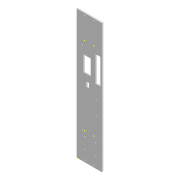
# Autodesk Inventor part: top of drivetrain 2
Saved by Autodesk Inventor 2020 (Build 240168000, 168)
## iProperties
Created: 2020-03-07
Part Number: top of drivetrain 2
Material: Generic
Document SubType Name: Modeling
Designer: jackm
Density: 1 g/cm^3
Appearance: Default
Author: jackm
Autodesk Inventor part; units mm, degrees
ref_plane "YZ Plane" through (0, 0, 0) normal (1, 0, 0) x (0, 1, 0)
ref_plane "XZ Plane" through (0, 0, 0) normal (0, 1, 0) x (-1, 0, 0)
ref_plane "XY Plane" through (0, 0, 0) normal (0, 0, 1) x (1, 0, 0)
ref_plane "Work Plane1" through (0, 0, 0) normal (0, 0, 1) x (0, -1, 0)
sketch "Sketch1" plane through (0, 0, 0) normal (0, 0, 1) x (0, -1, 0)
  line L0 (-450.85, 82.6732) -> (0, 82.6732) construction
  line L1 (0, -5) -> (-450.85, -5) construction
  line L2 (-450.85, -5) -> (-450.85, 82.6732)
  line L3 (0, 82.6732) -> (0, -5)
  line L4 (0, -5) -> (-450.85, -5)
  circle A0 centre (-444.5, 22.86) radius 1.7 construction
  circle A1 centre (-444.5, 54.8132) radius 1.7 construction
  circle A2 centre (-252.8255, 65.525) radius 1.9304 construction
  circle A3 centre (-210.0251, 65.525) radius 1.9304 construction
  circle A4 centre (-6.35, 54.8132) radius 1.7 construction
  circle A5 centre (-6.35, 22.86) radius 1.7 construction
  circle A6 centre (-94.9, 14.5) radius 1.7 construction
  circle A7 centre (-349.219, 14.5) radius 1.7 construction
  circle A8 centre (-444.5, 22.86) radius 1.7
  circle A9 centre (-444.5, 54.8132) radius 1.7
  circle A10 centre (-349.219, 14.5) radius 1.7
  circle A11 centre (-210.0251, 65.525) radius 1.7
  circle A12 centre (-94.9, 14.5) radius 1.7
  circle A13 centre (-6.35, 54.8132) radius 1.7
  circle A14 centre (-6.35, 22.86) radius 1.7
  circle A15 centre (-78.0653, 61.3428) radius 1.905
  line L5 (-78.0653, 61.3428) -> (-78.0653, 23.2428) construction
  line L6 (-78.0653, 23.2428) -> (-39.9653, 23.2428) construction
  line L7 (-39.9653, 23.2428) -> (-39.9653, 61.3428) construction
  circle A16 centre (-78.0653, 23.2428) radius 1.905
  circle A17 centre (-39.9653, 23.2428) radius 1.905
  circle A18 centre (-39.9653, 61.3428) radius 1.905
  line L8 (-450.85, 15.32) -> (-438.15, 15.32) construction
  line L9 (-246.7618, 27.8034) -> (-231.5218, 27.8034)
  line L10 (-231.5218, 27.8034) -> (-231.5218, 37.9634)
  line L11 (-231.5218, 37.9634) -> (-246.7618, 37.9634)
  line L12 (-246.7618, 37.9634) -> (-246.7618, 27.8034)
  line L13 (-345.7194, 77.136) -> (-345.7194, 60.0672)
  line L14 (-345.7194, 60.0672) -> (-256.8194, 60.0672)
  line L15 (-256.8194, 60.0672) -> (-256.8194, 77.136)
  line L16 (-450.85, 82.6732) -> (-345.7194, 82.6732)
  line L17 (-450.85, 82.6732) -> (0, 82.6732)
  circle A19 centre (-162.5271, 65.525) radius 1.7
  circle A20 centre (-244.1194, 68.6016) radius 1.1906
  line L18 (-345.7194, 77.136) -> (-256.8194, 77.136)
  circle A21 centre (-358.4194, 68.6016) radius 1.1906
  line L19 (-301.2694, 60.0672) -> (-301.2694, 77.136) construction
  line L20 (-323.85, 17.86) -> (-270.51, 17.86)
  line L21 (-270.51, 17.86) -> (-270.51, 43.26)
  line L22 (-270.51, 43.26) -> (-323.85, 43.26)
  line L23 (-323.85, 43.26) -> (-323.85, 17.86)
  circle A22 centre (-264.16, 30.56) radius 1.1906
  circle A23 centre (-330.2, 30.56) radius 1.1906
  point P0 (0, 0)
  dimension "M3Clearance" = 3.4
  dimension "d1" = 3.4
  dimension "d2" = 3.4
  dimension "d4" = 3.4
  dimension "d5" = 3.4
  dimension "d6" = 3.4
  dimension "d7" = 3.4
  dimension "Number6Clearance" = 3.81
  dimension "d9" = 38.1
  dimension "d10" = 38.1
  dimension "d11" = 38.1
  dimension "d12" = 3.81
  dimension "d13" = 3.81
  dimension "d14" = 3.81
  dimension "d21" = 12.7
  dimension "d22" = 20.32
  dimension "d24" = 15.24
  dimension "d25" = 10.16
  dimension "d26" = 22.606
  dimension "d36" = 3.4
  dimension "d37" = 47.498
  dimension "d38" = 17.1482
  dimension "d39" = 17.1482
  dimension "Number6WoodScrewPilot" = 2.3813
  dimension "d41" = 8.5344
  dimension "d42" = 12.7
  dimension "d43" = 5.5372
  dimension "d44" = 17.0688
  dimension "d45" = 2.3813
  dimension "d46" = 8.5344
  dimension "d47" = 12.7
  dimension "d48" = 149.5806
  dimension "d49" = 44.45
  dimension "d50" = 127
  dimension "d51" = 53.34
  dimension "d52" = 22.86
  dimension "d53" = 25.4
  dimension "d54" = 2.3813
  dimension "d55" = 12.7
  dimension "d56" = 6.35
  dimension "d57" = 2.3813
  dimension "d58" = 6.35
  dimension "d59" = 12.7
  constraints: 44 end point, 16 centre point, 13 perpendicular, 10 coincident, 5 equal length, 2 horizontal, 2 midpoint, 2 point on line, 2 vertical
  measures "M3Clearance" diameter of A8
  measures "d1" diameter of A9
  measures "d2" diameter of A10
  measures "d4" diameter of A11
  measures "d5" diameter of A12
  measures "d6" diameter of A13
  measures "d7" diameter of A14
  measures "Number6Clearance" diameter of A15
  measures "d9" distance of L5.start L5.end
  measures "d10" distance of L5.end L6.end
  measures "d11" distance of L6.end L7.end
  measures "d12" diameter of A16
  measures "d13" diameter of A17
  measures "d14" diameter of A18
  measures "d21" distance of L8.start L8.end
  measures "d22" distance between parallel lines of L1 L8
  measures "d24" distance of L11.end L10.end
  measures "d25" distance of L10.end L9.end
  measures "d26" distance of L16.end L13.end
  measures "d36" diameter of A19
  measures "d37" distance of A19.centre A3.centre
  measures "d38" distance from line of L17 A3.centre
  measures "d39" distance from line of L0 A19.centre
  measures "Number6WoodScrewPilot" diameter of A20
  measures "d41" distance from line of L14 A20.centre
  measures "d42" distance from line of A20.centre L15
  measures "d43" distance between parallel lines of L17 L18
  measures "d44" distance between parallel lines of L18 L14
  measures "d45" diameter of A21
  measures "d46" distance from line of L14 A21.centre
  measures "d47" distance from line of L13 A21.centre
  measures "d48" distance between parallel lines of L19 L2
  measures "d49" distance between parallel lines of L13 L19
  measures "d50" distance between parallel lines of L23 L2
  measures "d51" distance between parallel lines of L21 L23
  measures "d52" distance between parallel lines of L20 L1
  measures "d53" distance between parallel lines of L22 L20
  measures "d54" diameter of A22
  measures "d55" distance from line of A22.centre L20
  measures "d56" distance from line of A22.centre L21
  measures "d57" diameter of A23
  measures "d58" distance from line of L23 A23.centre
  measures "d59" distance from line of A23.centre L20
extrude "Extrusion1" add sketch "Sketch1" along normal blind 5
sketch "Sketch4" plane through (0, 0, 5) normal (0, 0, 1) x (1, 0, 0)
  circle A0 centre (54.8132, 95.25) radius 1.7 construction
  circle A1 centre (22.86, 95.25) radius 1.7 construction
  circle A2 centre (54.8132, 368.3) radius 1.7 construction
  circle A3 centre (22.86, 368.3) radius 1.7 construction
  circle A4 centre (22.86, 95.25) radius 1.7
  circle A5 centre (54.8132, 95.25) radius 1.7
  circle A6 centre (22.86, 368.3) radius 1.7
  circle A7 centre (54.8132, 368.3) radius 1.7
  point P0 (0, 0)
  dimension "d60" = 3.4
  dimension "d61" = 3.4
  dimension "d62" = 3.4
  dimension "d63" = 3.4
  constraints: 4 centre point, 4 coincident
  measures "d60" diameter of A4
  measures "d61" diameter of A5
  measures "d62" diameter of A6
  measures "d63" diameter of A7
extrude "Extrusion3" cut sketch "Sketch4" against normal blind 5
equation "\"d1\" = M3Clearance"
equation "\"d2\" = M3Clearance"
equation "\"d4\" = M3Clearance"
equation "\"d5\" = M3Clearance"
equation "\"d6\" = M3Clearance"
equation "\"d7\" = M3Clearance"
equation "\"d12\" = Number6Clearance"
equation "\"d13\" = Number6Clearance"
equation "\"d14\" = Number6Clearance"
equation "\"d21\" = d55"
equation "\"d36\" = M3Clearance"
equation "\"d39\" = d38"
equation "\"d41\" = 0.5 * d44"
equation "\"d45\" = Number6WoodScrewPilot"
equation "\"d46\" = d41"
equation "\"d47\" = d42"
equation "\"d54\" = Number6WoodScrewPilot"
equation "\"d55\" = 0.5 * d53"
equation "\"d57\" = Number6WoodScrewPilot"
equation "\"d58\" = d56"
equation "\"d60\" = M3Clearance"
equation "\"d61\" = M3Clearance"
equation "\"d62\" = M3Clearance"
equation "\"d63\" = M3Clearance"
body "Solid1"
